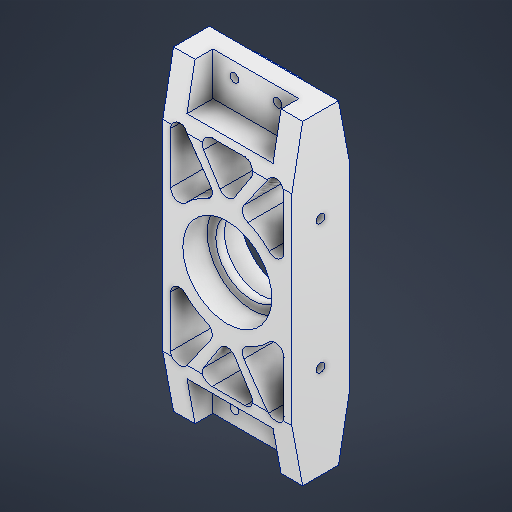
# Autodesk Inventor part: Suspension_Upright_V2
Saved by Autodesk Inventor 2026.1 (Build 301233000, 233)
## iProperties
Created: 2026-09-03
Part Number: Suspension_Upright_V2
Material: Aluminum 6061
Document SubType Name: Modeling
Designer: share
Density: 2.7 g/cm^3
Appearance: Aluminum - Flat
Mass: 1534.5 g
Surface Area: 680.642 cm^2
Volume: 568.332 cm^3
Author: share
Autodesk Inventor part; units mm, degrees
ref_plane "YZ Plane" through (0, 0, 0) normal (1, 0, 0) x (0, 1, 0)
ref_plane "XZ Plane" through (0, 0, 0) normal (0, 1, 0) x (-1, 0, 0)
ref_plane "XY Plane" through (0, 0, 0) normal (0, 0, 1) x (1, 0, 0)
sketch "Sketch1" plane through (0, 0, 0) normal (1, 0, 0) x (0, 1, 0)
  line L0 (-70, -20) -> (70, -20)
  line L1 (70, -20) -> (70, 20) construction
  line L2 (70, 20) -> (-70, 20)
  line L3 (-70, 20) -> (-70, -20) construction
  line L4 (0, 23.8) -> (0, -23.8) construction
  line L5 (-154, 0) -> (154, 0) construction
  line L6 (70, 20) -> (110, 12.5)
  line L7 (110, 12.5) -> (110, -12.5)
  line L8 (110, -12.5) -> (70, -20)
  line L9 (-70, 20) -> (-110, 12.5)
  line L10 (-110, 12.5) -> (-110, -12.5)
  line L11 (-110, -12.5) -> (-70, -20)
  point P0 (0, 0)
  dimension "d0" = 40
  dimension "d1" = 220
  dimension "d4" = 25
  dimension "d5" = 40
  constraints: 20 end point, 2 parallel, 2 symmetric about line, 1 equal length, 1 horizontal, 1 perpendicular, 1 vertical, 1 other
  measures "d0" distance between parallel lines of L0 L2
  measures "d1" distance between parallel lines of L10 L7
  measures "d4" distance of L9.end L10.end
  measures "d5" distance between parallel lines of L10 L3
extrude "Main Body" add sketch "Sketch1" along normal mid plane 90
sketch "Sketch2" plane through (-45, -70, 20) normal (0, 0, 1) x (1, 0, 0)
  circle A0 centre (45, 70) radius 25
  dimension "d8" = 50
  constraints: 1 centre point, 1 coincident
  measures "d8" diameter of A0
extrude "Center Bore" cut sketch "Sketch2" against normal through all
sketch "Sketch3" plane through (-45, -70, 20) normal (0, 0, 1) x (1, 0, 0)
  circle A0 centre (45, 70) radius 31
  circle A1 centre (45, 70) radius 25 projected
  dimension "d11" = 62
  constraints: 1 centre point, 1 coincident
  measures "d11" diameter of A0
extrude "Bearing Pocket 1" cut sketch "Sketch3" against normal blind 17
sketch "Sketch4" plane through (45, 70, -20) normal (0, 0, -1) x (-1, 0, 0)
  circle A0 centre (45, -70) radius 31 projected
  circle A1 centre (45, -70) radius 25 projected
extrude "Bearing Pocket 2" cut sketch "Sketch4" against normal blind 17
sketch "Sketch5" plane through (-45, -70, 20) normal (0, 0, 1) x (1, 0, 0)
  line L0 (75, 150) -> (15, 150)
  line L1 (45, 228) -> (45, -108) construction
  line L2 (-18, 70) -> (108, 70) construction
  line L3 (0, 180) -> (90, 180) projected
  line L4 (15, 150) -> (15, 180)
  line L5 (75, 150) -> (75, 180)
  line L6 (75, -10) -> (15, -10)
  line L7 (15, -10) -> (15, -40)
  line L8 (75, -10) -> (75, -40)
  line L9 (0, -40) -> (90, -40) projected
  point P0 (45, 70)
  dimension "d18" = 80
  dimension "d21" = 60
  constraints: 12 end point, 5 symmetric about line, 1 perpendicular, 1 point on line
  measures "d18" distance between parallel lines of L0 L2
  measures "d21" distance between parallel lines of L5 L4
extrude "R: Rod End Bracket Slots" cut sketch "Sketch5" against normal blind 20
sketch "Sketch6" plane through (-45, -70, 0) normal (0, 0, 1) x (1, 0, 0)
  line L0 (-18, 70) -> (108, 70) construction
  line L1 (15, 150) -> (15, 180) construction
  line L2 (75, 180) -> (75, 150) construction
  line L3 (45, 226) -> (45, -96) construction
  line L4 (30, 170) -> (60, 170) construction
  point P0 (45, 70)
  point P1 (30, -30)
  point P2 (60, -30)
  dimension "d26" = 30
  dimension "d27" = 200
  constraints: 3 symmetric about line, 2 end point, 1 horizontal, 1 parallel
  measures "d26" distance of L4.end L4.start
  measures "d27" distance from line of point (30, -30) L4
hole "R: Rod End Braket Mounting Holes" at (-15, 100, 0) at (15, 100, 0) at (-15, -100, 0) at (15, -100, 0) direction (0, 0, -1) diameter 6 end through all
sketch "Sketch8" plane through (-45, -70, 0) normal (0, 0, 1) x (1, 0, 0)
  circle A0 centre (30, 170) radius 3 projected
  circle A1 centre (60, 170) radius 3 projected
  arc A2 (30, 177.5) -> (30, 162.5) centre (30, 170) ccw
  arc A3 (60, 162.5) -> (60, 177.5) centre (60, 170) ccw
  line L0 (-18, 70) -> (108, 70) construction
  line L1 (30, 177.5) -> (60, 177.5)
  line L2 (30, 162.5) -> (60, 162.5)
  arc A4 (30, -22.5) -> (30, -37.5) centre (30, -30) ccw
  arc A5 (60, -37.5) -> (60, -22.5) centre (60, -30) ccw
  line L3 (30, -37.5) -> (60, -37.5)
  line L4 (30, -22.5) -> (60, -22.5)
  circle A6 centre (60, -30) radius 3 projected
  circle A7 centre (30, -30) radius 3 projected
  point P0 (45, 70)
  dimension "d37" = 15
  constraints: 8 end point, 8 point on circle, 6 symmetric about line, 4 centre point, 4 tangent, 2 coincident, 1 equal radius, 2 other
  measures "d37" distance between parallel lines of L2 L1
extrude "Rod End Bracket Nut Platforms" add sketch "Sketch8" against normal blind 15.7
sketch "Sketch9" plane through (-45, -70, 20) normal (0, 0, 1) x (1, 0, 0)
  circle A0 centre (45, 70) radius 40
  line L0 (45, 224) -> (45, -84) construction
  line L1 (-18, 70) -> (108, 70) construction
  line L2 (5.5, 76.3048) -> (5.5, 156.3048)
  line L3 (5.5, 156.3048) -> (38.3167, 109.4377)
  line L4 (84.5, 76.3048) -> (84.5, 156.3048)
  line L5 (84.5, 156.3048) -> (51.6833, 109.4377)
  line L6 (5.5, 63.6952) -> (5.5, -16.3048)
  line L7 (5.5, -16.3048) -> (38.3167, 30.5623)
  line L8 (84.5, 63.6952) -> (84.5, -16.3048)
  line L9 (84.5, -16.3048) -> (51.6833, 30.5623)
  line L10 (45, 110) -> (22.5, 145)
  line L11 (22.5, 145) -> (67.5, 145)
  line L12 (67.5, 145) -> (45, 110)
  line L13 (45, 30) -> (22.5, -5)
  line L14 (22.5, -5) -> (67.5, -5)
  line L15 (67.5, -5) -> (45, 30)
  point P0 (84.5, 76.3048)
  point P1 (84.5, 63.6952)
  point P2 (85, 70)
  point P3 (51.6833, 109.4377)
  point P4 (51.6833, 30.5623)
  point P5 (5.5, 63.6952)
  point P6 (5, 70)
  point P7 (38.3167, 30.5623)
  dimension "d40" = 80
  dimension "d41" = 80
  dimension "d43" = 35
  dimension "d44" = 35
  dimension "d45" = 45
  dimension "d48" = 79
  constraints: 28 end point, 12 symmetric about line, 3 point on circle, 1 centre point, 1 coincident, 1 horizontal, 1 point on line, 1 vertical, 1 other
  measures "d40" diameter of A0
  measures "d41" distance of L2.start L2.end
  measures "d43" angle of L3 L2
  measures "d44" distance from line of L10.start L11
  measures "d45" distance of L10.end L11.end
  measures "d48" distance between parallel lines of L4 L2
extrude "Weight Reduction Pockets" cut sketch "Sketch9" against normal through all contours L15 L14 L13 | L10 L11 L12 | A0 L5 L4 | L8 L9 A0 | A0 L2 L3 | L7 L6 A0
fillet "Weight Reduction Fillets" radius 6 18 edges at (39.5, -6.3048, 0) (39.5, 6.3048, 0) (-39.5, 6.3048, 0) (-39.5, -6.3048, 0) (-6.6833, -39.4377, 0) (6.6833, -39.4377, 0) (0, -40, 0) (0, 40, 0) (-6.6833, 39.4377, 0) (6.6833, 39.4377, 0) (-39.5, -86.3048, 0) (-22.5, -75, 0) (22.5, -75, 0) (39.5, -86.3048, 0) (-39.5, 86.3048, 0) (39.5, 86.3048, 0) (-22.5, 75, 0) (22.5, 75, 0)
sketch "Sketch10" plane through (-45, 0, 0) normal (-1, 0, 0) x (0, 0, 1)
  line L0 (0, 154) -> (0, -154) projected
  line L1 (-28, 0) -> (28, 0) projected
  point P0 (0, 0)
  point P1 (0, -45)
  point P2 (0, 45)
  dimension "d55" = 90
  constraints: 2 point on line, 1 symmetric about line
  measures "d55" distance of point (0, 45) point (0, -45)
hole "R: Brake Caliper Bracket Holes" at (-45, -45, 0) at (-45, 45, 0) direction (1, 0, 0) diameter 6 depth 5.5 tip angle 118
sketch "Sketch11" plane through (45, 0, 0) normal (1, 0, 0) x (0, 0, -1)
  line L0 (-28, 0) -> (28, 0) construction
  line L1 (0, -154) -> (0, 154) construction
  point P0 (0, 0)
  point P1 (0, -45)
  point P2 (0, 45)
  dimension "d63" = 90
  constraints: 2 point on line, 1 symmetric about line
  measures "d63" distance of point (0, 45) point (0, -45)
hole "L: Brake Caliper Bracket Holes" at (45, -45, 0) at (45, 45, 0) direction (-1, 0, 0) diameter 6 depth 5.5 tip angle 118
equation "\"Main_Body_Height\" = 1"
equation "\"Main_Body_Diagonal\" = 1"
equation "\"Main_Body_Thickness\" = 1"
equation "\"Main_Body_Tip_Width\" = 1"
equation "\"Bearing_Bore_Depth\" = 1"
body "Solid1"
